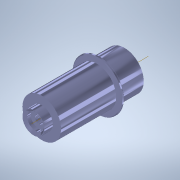
# Autodesk Inventor part: shocks_spring
Saved by Autodesk Inventor 2020 (Build 240168000, 168)
## iProperties
Created: 2015-12-01
Part Number: shocks_spring
Material: Plata
Document SubType Name: Modeling
Designer: MIGUEL ANGEL
Density: 10.49 g/cm^3
Appearance: Cromo - Azul Pulido
Author: MIGUEL ANGEL
Autodesk Inventor part; units mm, degrees
ref_plane "YZ Plane" through (0, 0, 0) normal (1, 0, 0) x (0, 1, 0)
ref_plane "XZ Plane" through (0, 0, 0) normal (0, 1, 0) x (-1, 0, 0)
ref_plane "XY Plane" through (0, 0, 0) normal (0, 0, 1) x (1, 0, 0)
sketch "Boceto1" plane through (0, 0, 0) normal (0, 1, 0) x (-1, 0, 0)
  circle A0 centre (0, 0) radius 14
  dimension "d0" = 28
  constraints: 1 centre point, 1 coincident
  measures "d0" diameter of A0
extrude "Extrusión1" add sketch "Boceto1" along normal blind 60
shell "Vaciado1" thickness 2 removed faces 1 at (-2.651, 60, 3.8406)
sketch "Boceto2" plane through (0, 0, 0) normal (1, 0, 0) x (0, 1, 0)
  line L0 (0, -14) -> (60, -14) projected
  line L1 (0, 14) -> (60, 14) projected
  line L2 (46, -14) -> (48, -14)
  line L3 (48, -14) -> (48, -19)
  line L4 (48, -19) -> (46, -19)
  line L5 (46, -19) -> (46, -14)
  point P0 (0, 0)
  dimension "d4" = 14
  dimension "d5" = 2
  dimension "d6" = 5
  constraints: 8 end point, 2 parallel, 1 horizontal, 1 perpendicular, 1 point on line
  measures "d4" distance from line of L0.end L5
  measures "d5" distance between parallel lines of L5 L3
  measures "d6" distance between parallel lines of L0 L4
sketch "Boceto3" plane through (0, 0, 0) normal (1, 0, 0) x (0, 1, 0)
  line L0 (84.0119, 0) -> (36.1853, 0)
  point P0 (0, 0)
  constraints: 2 end point, 1 horizontal
sketch "Boceto4" plane through (0, 0, 0) normal (0, -1, 0) x (1, 0, 0)
  circle A0 centre (0, 0) radius 3
  circle A1 centre (0, 0) radius 6
  dimension "d7" = 6
  dimension "d8" = 12
  constraints: 2 centre point, 2 coincident
  measures "d7" diameter of A0
  measures "d8" diameter of A1
extrude "Extrusión2" cut sketch "Boceto4" against normal through all contours A0
sketch "Boceto5" plane through (0, 0, 0) normal (0, -1, 0) x (1, 0, 0)
  circle A0 centre (0, 0) radius 3 projected
sketch "Boceto6" plane through (0, 0, 0) normal (0, 0, 1) x (1, 0, 0)
  line L0 (-14, 0) -> (-14, 60) projected
  line L1 (-14, 42) -> (-18, 42)
  line L2 (-18, 42) -> (-18, 40)
  line L3 (-18, 40) -> (-14, 40)
  line L4 (14, 60) -> (-14, 60) projected
  line L5 (0, -14.2107) -> (0, 116.483)
  point P0 (0, 0)
  dimension "d11" = 18
  dimension "d12" = 2
  dimension "d13" = 4
  constraints: 8 end point, 3 perpendicular, 2 point on line, 1 vertical
  measures "d11" distance between parallel lines of L4 L1
  measures "d12" distance between parallel lines of L1 L3
  measures "d13" distance between parallel lines of L0 L2
sketch "Boceto7" plane through (0, 0, 0) normal (0, -1, 0) x (1, 0, 0)
  circle A0 centre (0, 0) radius 3 projected
  circle A1 centre (0, 0) radius 8
  dimension "d14" = 16
  constraints: 1 centre point, 1 coincident
  measures "d14" diameter of A1
extrude "Extrusión3" add sketch "Boceto7" along normal blind 6
sketch "Boceto8" plane through (0, -6, 0) normal (0, -1, 0) x (1, 0, 0)
  circle A0 centre (0, 0) radius 8 projected
  circle A1 centre (0, 0) radius 6
  circle A2 centre (0, 0) radius 3 projected
  dimension "d17" = 2
  constraints: 1 centre point
  measures "d17" radial gap between concentric circles of A0 A1
extrude "Extrusión4" cut sketch "Boceto8" against normal blind 4 contours A1
chamfer "Chaflán1" distance 1.5 angle 45 1 edges at (-6, -6, 0)
revolve "Revolución1" add sketch "Boceto6" angle 360 about axis through (0, -14.2107, 0) along (0, 1, 0)
chamfer "Chaflán2" distance 0.5 angle 45 2 edges at (18, 40, 0) (18, 42, 0)
